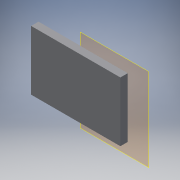
# Autodesk Inventor part: Part Plate
Saved by Autodesk Inventor 2016 (Build 200138000, 138)
## iProperties
Created: 2016-04-23
Part Number: Part Plate
Material: Generic
Document SubType Name: Modeling
Designer: Scott
Density: 1 g/cm^3
Appearance: Default
Author: Scott
Autodesk Inventor part; units mm, degrees
ref_plane "YZ Plane" through (0, 0, 0) normal (1, 0, 0) x (0, 1, 0)
ref_plane "XZ Plane" through (0, 0, 0) normal (0, 1, 0) x (-1, 0, 0)
ref_plane "XY Plane" through (0, 0, 0) normal (0, 0, 1) x (1, 0, 0)
ref_plane "Work Plane1" through (0, 0, 0) normal (0, 0, 1) x (1, 0, 0)
sketch "Sketch1" plane through (0, 0, 0) normal (0, 0, 1) x (1, 0, 0)
  line L0 (-288.275, -58.41) -> (-48.275, -58.41)
  line L1 (-48.275, -58.41) -> (-48.275, 101.59)
  line L2 (-48.275, 101.59) -> (-288.275, 101.59)
  line L3 (-288.275, 101.59) -> (-288.275, -58.41)
  line L4 (-288.275, -58.41) -> (-48.275, 101.59) construction
  line L5 (-48.275, -58.41) -> (-288.275, 101.59) construction
  point P0 (0, 0)
  point P1 (-168.275, 21.59)
  dimension "d0" = 240
  dimension "d1" = 160
  constraints: 12 end point, 2 midpoint, 2 parallel, 1 horizontal, 1 perpendicular
  measures "d0" distance of L2.end L1.end
  measures "d1" distance of L1.end L0.end
extrude "Extrusion1" add sketch "Sketch1" along normal blind 20
body "Solid1"
